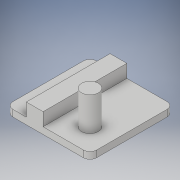
# Autodesk Inventor part: tapa_canyon_cambio
Saved by Autodesk Inventor 2019 (Build 230136000, 136)
## iProperties
Created: 2019-01-03
Part Number: tapa_canyon_cambio
Material: Generic
Document SubType Name: Modeling
Designer: assman
Density: 1 g/cm^3
Appearance: Default
Author: assman
## iProperties of the stored document tapa_canyon_cambio_3DPrint.ipt
Created: 2019-01-03
Part Number: tapa_canyon_cambio_3DPrint
Material: Generic
Document SubType Name: Modeling
Designer: assman
Density: 1 g/cm^3
Appearance: Default
Author: assman
Autodesk Inventor part; units mm, degrees
ref_plane "YZ Plane" through (0, 0, 0) normal (1, 0, 0) x (0, 1, 0)
ref_plane "XZ Plane" through (0, 0, 0) normal (0, 1, 0) x (-1, 0, 0)
ref_plane "XY Plane" through (0, 0, 0) normal (0, 0, 1) x (1, 0, 0)
sketch "Sketch1" plane through (0, 0, 0) normal (0, 1, 0) x (-1, 0, 0)
  line L0 (0, 0) -> (25, 0)
  line L1 (25, 0) -> (25, -25)
  line L2 (25, -25) -> (0, -25)
  line L3 (0, -25) -> (0, 0)
  dimension "d0" = 25
  dimension "d1" = 25
  constraints: 8 end point, 2 parallel, 1 coincident, 1 horizontal, 1 perpendicular
  measures "d0" distance of L1.end L2.end
  measures "d1" distance of L0.end L1.end
extrude "Extrusion1" add sketch "Sketch1" along normal blind 2
fillet "Fillet1" radius 2 4 edges at (0, 1, 0) (0, 1, -25) (-25, 1, 0) (-25, 1, -25)
sketch "Sketch2" plane through (0, 2, 0) normal (0, 1, 0) x (1, 0, 0)
  line L0 (-19, 25) -> (-19, 0)
  line L1 (-25, 23) -> (-25, 2) projected
  line L2 (-14, 25) -> (-14, 0)
  line L3 (-19, 25) -> (-14, 25)
  line L4 (-2, 25) -> (-23, 25) projected
  line L5 (-19, 0) -> (-14, 0)
  line L6 (-23, 0) -> (-2, 0) projected
  point P0 (0, 0)
  dimension "d5" = 6
  dimension "d6" = 5
  constraints: 8 end point, 2 collinear, 2 vertical
  measures "d5" distance between parallel lines of L1 L0
  measures "d6" distance between parallel lines of L0 L2
extrude "Extrusion2" add sketch "Sketch2" along normal blind 3.9
sketch "Sketch4" plane through (0, 2, 0) normal (0, 1, 0) x (1, 0, 0)
  line L0 (-2, 25) -> (-14, 25) projected
  line L1 (0, 2) -> (0, 23) projected
  circle A0 centre (-7, 7) radius 2.5
  line L2 (-14, 0) -> (-2, 0) projected
  point P0 (0, 0)
  dimension "d11" = 5
  dimension "d14" = 7
  dimension "d15" = 7
  constraints: 1 centre point, 1 coincident
  measures "d11" diameter of A0
  measures "d14" distance from line of L2 A0.centre
  measures "d15" distance from line of L1 A0.centre
extrude "Extrusion3" add sketch "Sketch4" along normal blind 10
body "Solid1"
